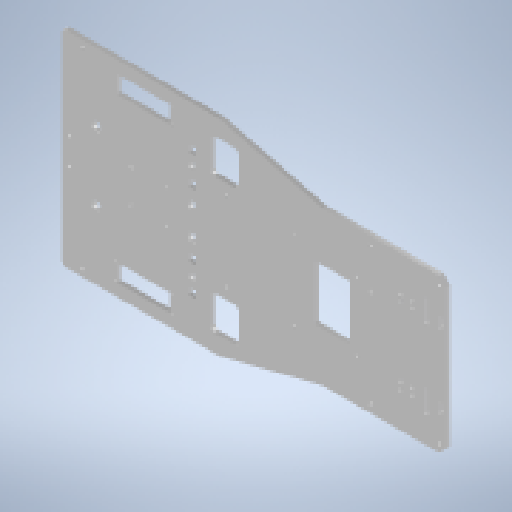
# Autodesk Inventor part: Base3
Saved by Autodesk Inventor 2023 (Build 270158000, 158)
## iProperties
Created: 2023-12-01
Part Number: Base3
Material: Aluminio 6061
Document SubType Name: Modeling
Designer: ASUS
Density: 2.7 g/cm^3
Appearance: Aluminio - Plano
Author: ASUS
Autodesk Inventor part; units mm, degrees
ref_plane "YZ Plane" through (0, 0, 0) normal (1, 0, 0) x (0, 1, 0)
ref_plane "XZ Plane" through (0, 0, 0) normal (0, 1, 0) x (-1, 0, 0)
ref_plane "XY Plane" through (0, 0, 0) normal (0, 0, 1) x (1, 0, 0)
sketch "Boceto1" plane through (0, 0, 0) normal (0, 0, 1) x (1, 0, 0)
  line L0 (-200, -75) -> (-85, -75)
  line L1 (-85, -75) -> (-10.0003, -56)
  line L2 (-200, 75) -> (-200, -75)
  line L3 (-84.9998, 75) -> (-200, 75)
  line L4 (75, -56) -> (-10.0003, -56)
  line L5 (80, -51) -> (80, 50.9899)
  line L6 (75, -56) -> (80, -51)
  line L7 (80, 50.9899) -> (75, 56)
  line L8 (75, 56) -> (-10, 56)
  arc A0 (-200, -72) -> (-197, -75) centre (-197, -72) ccw
  arc A1 (-197, 75) -> (-200, 72) centre (-197, 72) ccw
  line L9 (-16, 20) -> (10, 20)
  line L10 (10, -20) -> (10, 20)
  line L11 (-16, -20) -> (10, -20)
  line L12 (-16, -20) -> (-16, 20)
  line L13 (-160, -53.1464) -> (-121.4, -53.1464)
  line L14 (-121.4, -53.1464) -> (-121.4, -65.7464)
  line L15 (-160, -65.7464) -> (-121.4, -65.7464)
  line L16 (-160, -65.7464) -> (-160, -53.1464)
  line L17 (-88, -37) -> (-74, -37)
  line L18 (-91, -59) -> (-91, -40)
  line L19 (-71, -40) -> (-71, -59)
  line L20 (-74, -62) -> (-88, -62)
  line L21 (-121.4, 65.7464) -> (-160, 65.7464)
  line L22 (-160, 53.1464) -> (-160, 65.7464)
  line L23 (-121.4, 53.1464) -> (-160, 53.1464)
  line L24 (-121.4, 65.7464) -> (-121.4, 53.1464)
  line L25 (-88, 62) -> (-74, 62)
  line L26 (-91, 40) -> (-91, 59)
  line L27 (-74, 37) -> (-88, 37)
  line L28 (-71, 59) -> (-71, 40)
  arc A2 (-91, -59) -> (-88, -62) centre (-88, -59) ccw
  arc A3 (-74, -62) -> (-71, -59) centre (-74, -59) ccw
  arc A4 (-71, -40) -> (-74, -37) centre (-74, -40) ccw
  arc A5 (-88, -37) -> (-91, -40) centre (-88, -40) ccw
  arc A6 (-74, 37) -> (-71, 40) centre (-74, 40) ccw
  arc A7 (-91, 40) -> (-88, 37) centre (-88, 40) ccw
  arc A8 (-88, 62) -> (-91, 59) centre (-88, 59) ccw
  arc A9 (-71, 59) -> (-74, 62) centre (-74, 59) ccw
  line L29 (-107.875, -47.5) -> (-102.125, -47.5)
  line L30 (-102.125, -42.5) -> (-102.125, -47.5)
  line L31 (-107.875, -47.5) -> (-107.875, -42.5)
  line L32 (-107.875, -42.5) -> (-102.125, -42.5)
  circle A10 centre (-105, -35) radius 2.5
  line L33 (-107.875, -26) -> (-102.125, -26)
  line L34 (-102.125, -21) -> (-102.125, -26)
  line L35 (-102.125, -21) -> (-107.875, -21)
  line L36 (-107.875, -21) -> (-107.875, -26)
  circle A11 centre (-105, -10) radius 3
  circle A12 centre (-124, -12) radius 1
  circle A13 centre (-150, -12) radius 1
  line L37 (-172.375, -23.2139) -> (-172.375, -26.7861)
  circle A14 centre (-175, -25) radius 3.175
  circle A15 centre (-119.7, -53.4464) radius 0.75
  circle A16 centre (-119.7, -65.4464) radius 0.75
  circle A17 centre (-161.7, -53.4464) radius 0.75
  circle A18 centre (-161.7, -65.4464) radius 0.75
  circle A19 centre (-184.9999, -70) radius 1.5
  circle A20 centre (-194.5, -10) radius 1.5
  circle A21 centre (-80, -29) radius 1.25
  circle A22 centre (-31, -29) radius 1.25
  circle A23 centre (24.9743, -49.9788) radius 1.5
  circle A24 centre (55, -30) radius 1.5
  circle A25 centre (55, -25) radius 1.5
  circle A26 centre (47, -25) radius 1.5
  circle A27 centre (47, -30) radius 1.5
  circle A28 centre (15.0745, -24.9255) radius 1.5
  line L38 (80, -0.0035) -> (-200, 0.0684) construction
  line L39 (-107.8506, 47.5895) -> (-102.1006, 47.5865)
  line L40 (-102.1031, 42.5865) -> (-102.1006, 47.5865)
  line L41 (-107.8506, 47.5895) -> (-107.8531, 42.5895)
  line L42 (-107.8531, 42.5895) -> (-102.1031, 42.5865)
  circle A29 centre (-104.982, 35.088) radius 2.5
  line L43 (-107.8616, 26.0895) -> (-102.1116, 26.0865)
  line L44 (-102.1142, 21.0865) -> (-102.1116, 26.0865)
  line L45 (-102.1142, 21.0865) -> (-107.8642, 21.0895)
  line L46 (-107.8642, 21.0895) -> (-107.8616, 26.0895)
  circle A30 centre (-104.9948, 10.088) radius 3
  circle A31 centre (-123.9938, 12.0978) radius 1
  circle A32 centre (-149.9938, 12.1111) radius 1
  line L47 (-172.363, 23.3366) -> (-172.3612, 26.9087)
  circle A33 centre (-174.9871, 25.124) radius 3.175
  circle A34 centre (-119.6725, 53.542) radius 0.75
  circle A35 centre (-119.6663, 65.5419) radius 0.75
  circle A36 centre (-184.9639, 70.1291) radius 1.5
  circle A37 centre (-194.4948, 10.134) radius 1.5
  circle A38 centre (-79.9851, 29.0752) radius 1.25
  circle A39 centre (-30.9851, 29.05) radius 1.25
  circle A40 centre (25, 50) radius 1.5
  circle A41 centre (55.0154, 30.0058) radius 1.5
  circle A42 centre (55.0129, 25.0058) radius 1.5
  circle A43 centre (47.0129, 25.0099) radius 1.5
  circle A44 centre (47.0155, 30.0098) radius 1.5
  circle A45 centre (15.0873, 24.9518) radius 1.5
  line L48 (-10, 56) -> (-85, 75.0001)
  line L49 (-200, 75) -> (80, 75)
  line L50 (80, 75) -> (80, -75)
  line L51 (80, -75) -> (-200, -75)
  line L52 (-200, -75) -> (-200, 75)
  line L53 (65.4, 19.7) -> (65.4, 37.2) construction
  line L54 (66.9, 21.2) -> (66.9, 35.7)
  line L55 (63.9, 35.7) -> (63.9, 21.2)
  arc A46 (63.9, 21.2) -> (66.9, 21.2) centre (65.4, 21.2) ccw
  arc A47 (66.9, 35.7) -> (63.9, 35.7) centre (65.4, 35.7) ccw
  line L56 (76.2, -22.755) -> (76.2, 22.745) construction
  line L57 (76.2, 22.745) -> (76.2, 31.045) construction
  line L58 (77.5, 24.045) -> (77.5, 29.745)
  line L59 (74.9, 29.745) -> (74.9, 24.045)
  arc A48 (74.9, 24.045) -> (77.5, 24.045) centre (76.2, 24.045) ccw
  arc A49 (77.5, 29.745) -> (74.9, 29.745) centre (76.2, 29.745) ccw
  line L60 (65.3899, -19.6996) -> (65.3809, -37.1996) construction
  line L61 (66.8891, -21.2004) -> (66.8816, -35.7004)
  line L62 (63.8816, -35.6988) -> (63.8891, -21.1988)
  arc A50 (66.8891, -21.2004) -> (63.8891, -21.1988) centre (65.3891, -21.1996) ccw
  arc A51 (63.8816, -35.6988) -> (66.8816, -35.7004) centre (65.3816, -35.6996) ccw
  line L63 (76.1883, -22.7501) -> (76.184, -31.0501) construction
  line L64 (77.4876, -24.0508) -> (77.4847, -29.7508)
  line L65 (74.8847, -29.7494) -> (74.8876, -24.0494)
  arc A52 (77.4876, -24.0508) -> (74.8876, -24.0494) centre (76.1876, -24.0501) ccw
  arc A53 (74.8847, -29.7494) -> (77.4847, -29.7508) centre (76.1847, -29.7501) ccw
  circle A54 centre (75, -50) radius 1.25
  circle A55 centre (75, 50) radius 1.25
  circle A56 centre (25, 21) radius 1.5
  point P0 (-91, -37)
  point P1 (-71, 37)
  point P2 (-91, -62)
  point P3 (-121.4, 62)
  point P4 (80, -51)
  point P5 (-85, -75)
  point P6 (65.4, 28.45)
  point P7 (76.2, -0.005)
  point P8 (80, -0.005)
  point P9 (76.2, 26.895)
  point P10 (65.3854, -28.4496)
  point P11 (76.1862, -26.9001)
  dimension "d24" = 3
  dimension "d25" = 3
  dimension "d26" = 3
  dimension "d28" = 17.5
  dimension "d29" = 18.8
  dimension "d30" = 3
  dimension "d32" = 45.5
  dimension "d33" = 8.3
  dimension "d34" = 2.6
  dimension "d35" = 3
  dimension "d36" = 35
  dimension "d37" = 2.5
  dimension "d38" = 8
  constraints: 140 end point, 55 centre point, 46 symmetric about line, 45 point on circle, 26 point on line, 8 tangent, 4 midpoint, 4 parallel, 4 vertical, 2 horizontal, 1 horizontal alignment, 1 perpendicular, 26 other
  measures "d24" radius of A0
  measures "d25" radius of A2
  measures "d26" radius of A8
  measures "d28" distance of L53.start L53.end
  measures "d29" distance from line of L8 L53.end
  measures "d30" distance between parallel lines of L54 L55
  measures "d32" distance of L56.start L56.end
  measures "d33" distance of L56.end L57.end
  measures "d34" diameter of A49
  measures "d35" diameter of A56
  measures "d36" distance from line of L8 A56.centre
  measures "d37" distance between parallel lines of L5 L58
  measures "d38" distance between parallel lines of L59 L54
extrude "Extrusión1" add sketch "Boceto1" along normal blind 3 contours A0 L2 A1 L3 L48 L8 L7 L5 L6 L4 L1 L0
